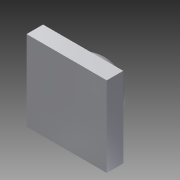
# Autodesk Inventor part: PowerLED
Saved by Autodesk Inventor 2013 (Build 170138000, 138)
## iProperties
Created: 2015-07-04
Part Number: PowerLED
Material: Szkło, lane, przezroczyste
Document SubType Name: Modeling
Designer: terg
Density: 1 g/cm^3
Author: terg
Autodesk Inventor part; units mm, degrees
ref_plane "YZ Plane" through (0, 0, 0) normal (1, 0, 0) x (0, 1, 0)
ref_plane "XZ Plane" through (0, 0, 0) normal (0, 1, 0) x (-1, 0, 0)
ref_plane "XY Plane" through (0, 0, 0) normal (0, 0, 1) x (1, 0, 0)
sketch "Szkic1" plane through (0, 0, 0) normal (0, 1, 0) x (-1, 0, 0)
  line L0 (0, 0) -> (3.45, 0)
  line L1 (3.45, 0) -> (3.45, 3.45)
  line L2 (3.45, 3.45) -> (0, 3.45)
  line L3 (0, 3.45) -> (0, 0)
  dimension "d0" = 3.45
  dimension "d1" = 3.45
  constraints: 8 end point, 2 parallel, 1 horizontal, 1 perpendicular
  measures "d0" distance of L2.end L1.end
  measures "d1" distance of L1.end L0.end
extrude "Wyciągnięcie proste1" add sketch "Szkic1" along normal blind 0.71
sketch "Szkic2" plane through (0, 0.71, 0) normal (0, 1, 0) x (1, 0, 0)
  line L0 (0, 0) -> (-3.45, 0) projected
  line L1 (-3.45, 0) -> (-3.45, -3.45) projected
  line L2 (-3.45, -3.45) -> (0, -3.45) projected
  line L3 (0, -3.45) -> (0, 0) projected
  line L4 (-3.325, -0.125) -> (-2.925, -0.125)
  line L5 (-2.925, -0.125) -> (-2.925, -3.325)
  line L6 (-2.925, -3.325) -> (-3.325, -3.325)
  line L7 (-3.325, -3.325) -> (-3.325, -0.125)
  line L8 (-0.525, -0.125) -> (-0.125, -0.125)
  line L9 (-0.125, -0.125) -> (-0.125, -3.325)
  line L10 (-0.125, -3.325) -> (-0.525, -3.325)
  line L11 (-0.525, -3.325) -> (-0.525, -0.125)
  line L12 (-0.425, -0.525) -> (-0.225, -0.525)
  line L13 (-0.225, -0.525) -> (-0.225, -0.925)
  line L14 (-0.225, -0.925) -> (-0.425, -0.925)
  line L15 (-0.425, -0.925) -> (-0.425, -0.525)
  line L16 (-0.225, -2.525) -> (-0.425, -2.525)
  line L17 (-0.425, -2.525) -> (-0.425, -2.925)
  line L18 (-0.425, -2.925) -> (-0.225, -2.925)
  line L19 (-0.225, -2.925) -> (-0.225, -2.525)
  line L20 (-0.525, -0.425) -> (-1.425, -0.425)
  line L21 (-1.425, -0.425) -> (-1.425, -0.625)
  line L22 (-1.425, -0.625) -> (-0.525, -0.625)
  line L23 (-0.525, -0.625) -> (-0.525, -0.425)
  line L24 (-2.925, -0.425) -> (-2.025, -0.425)
  line L25 (-2.025, -0.425) -> (-2.025, -0.625)
  line L26 (-2.025, -0.625) -> (-2.925, -0.625)
  line L27 (-2.925, -0.625) -> (-2.925, -0.425)
  dimension "d4" = 0.4
  dimension "d5" = 3.2
  dimension "d6" = 0.125
  dimension "d7" = 0.125
  dimension "d8" = 0.125
  dimension "d9" = 0.4
  dimension "d10" = 3.2
  dimension "d11" = 0.125
  dimension "d12" = 0.125
  dimension "d13" = 0.2
  dimension "d14" = 0.4
  dimension "d15" = 0.2
  dimension "d16" = 0.4
  dimension "d17" = 0
  dimension "d18" = 0.1
  dimension "d19" = 0.1
  dimension "d20" = 0.4
  dimension "d21" = 0.4
  dimension "d22" = 0.9
  dimension "d23" = 0.2
  dimension "d24" = 0.1
  dimension "d25" = 0.1
  dimension "d26" = 0.9
  dimension "d27" = 0.2
  dimension "d28" = 0
  constraints: 48 end point, 12 parallel, 6 horizontal, 6 perpendicular, 2 point on line
  measures "d4" distance of L5.end L6.end
  measures "d5" distance of L4.end L5.end
  measures "d6" distance between parallel lines of L0 L4
  measures "d7" distance between parallel lines of L2 L6
  measures "d8" distance between parallel lines of L1 L7
  measures "d9" distance of L9.end L10.end
  measures "d10" distance of L8.end L9.end
  measures "d11" distance between parallel lines of L2 L10
  measures "d12" distance between parallel lines of L3 L9
  measures "d13" distance of L13.end L14.end
  measures "d14" distance of L12.end L13.end
  measures "d15" distance of L18.end L17.end
  measures "d16" distance of L17.end L16.end
  measures "d17" distance between parallel lines of L19 L13
  measures "d18" distance between parallel lines of L9 L13
  measures "d19" distance between parallel lines of L11 L15
  measures "d20" distance between parallel lines of L8 L12
  measures "d21" distance between parallel lines of L10 L18
  measures "d22" distance of L22.end L21.end
  measures "d23" distance of L21.end L20.end
  measures "d24" distance between parallel lines of L12 L22
  measures "d25" distance between parallel lines of L20 L12
  measures "d26" distance of L25.end L26.end
  measures "d27" distance of L24.end L25.end
  measures "d28" distance between parallel lines of L20 L24
extrude "Wyciągnięcie proste2" add sketch "Szkic2" along normal blind 0.01 contours L4 L5 L6 L7 | L24 L25 L26 L5 | L8 L9 L10 L11 | L11 L22 L21 L20
sketch "Szkic3" plane through (0, 0.71, 0) normal (0, 1, 0) x (1, 0, 0)
  line L0 (-3.45, 0) -> (-3.45, -3.45) projected
  line L1 (-3.45, -3.45) -> (0, -3.45) projected
  line L2 (0, -3.45) -> (0, 0) projected
  circle A0 centre (-1.725, -1.725) radius 1.3
  dimension "d31" = 1.725
  dimension "d32" = 1.725
  dimension "d33" = 1.725
  dimension "d34" = 2.6
  constraints: 1 centre point, 1 coincident
  measures "d31" distance from line of L2 point (-1.725, -1.725)
  measures "d32" distance from line of L0 point (-1.725, -1.725)
  measures "d33" distance from line of L1 point (-1.725, -1.725)
  measures "d34" diameter of A0
extrude "Wyciągnięcie proste3" add sketch "Szkic3" along normal blind 1.3
fillet "Zaokrąglenie1" radius 1.3 1 edges at (-3.025, 2.01, 1.725)
sketch "Szkic4" plane through (0, 0.71, 0) normal (0, 1, 0) x (1, 0, 0)
  arc A0 (-2.925, -2.225) -> (-0.525, -2.225) centre (-1.725, -1.725) ccw projected
  arc A1 (-1.425, -0.4601) -> (-2.025, -0.4601) centre (-1.725, -1.725) ccw projected
  line L0 (-2.43, -1.02) -> (-1.02, -1.02)
  line L1 (-1.02, -1.02) -> (-1.02, -2.43)
  line L2 (-1.02, -2.43) -> (-2.43, -2.43)
  line L3 (-2.43, -2.43) -> (-2.43, -1.02)
  dimension "d38" = 1.41
  dimension "d39" = 1.41
  dimension "d40" = 0.705
  dimension "d41" = 0.705
  constraints: 8 end point, 2 parallel, 1 horizontal, 1 perpendicular
  measures "d38" distance of L1.end L2.end
  measures "d39" distance of L0.end L1.end
  measures "d40" distance from line of A0.centre L1
  measures "d41" distance from line of A1.centre L0
extrude "Wyciągnięcie proste4" cut sketch "Szkic4" along normal blind 0.2
sketch "Szkic5" plane through (0, 0.71, 0) normal (0, 1, 0) x (1, 0, 0)
  line L0 (-2.42, -1.04) -> (-1.02, -1.04)
  line L1 (-1.02, -1.04) -> (-1.02, -2.44)
  line L2 (-1.02, -2.44) -> (-2.42, -2.44)
  line L3 (-2.42, -2.44) -> (-2.42, -1.04)
  line L4 (-2.43, -1.02) -> (-2.43, -2.43) projected
  line L5 (-2.43, -2.43) -> (-1.02, -2.43) projected
  dimension "d44" = 1.4
  dimension "d45" = 1.4
  dimension "d46" = 0.01
  dimension "d47" = 0.01
  constraints: 8 end point, 2 parallel, 1 horizontal, 1 perpendicular
  measures "d44" distance of L1.end L2.end
  measures "d45" distance of L0.end L1.end
  measures "d46" distance between parallel lines of L3 L4
  measures "d47" distance between parallel lines of L2 L5
extrude "Wyciągnięcie proste5" add sketch "Szkic5" along normal blind 0.19
equation "\"d6\" = d7"
equation "\"d8\" = d7"
equation "\"d9\" = d4"
equation "\"d10\" = d5"
equation "\"d11\" = d7"
equation "\"d12\" = d7"
equation "\"d18\" = d19"
equation "\"d21\" = d20"
equation "\"d24\" = d25"
equation "\"d31\" = d32"
equation "\"d33\" = d31"
equation "\"d40\" = 0.5 * d38"
equation "\"d41\" = 0.5 * d39"
